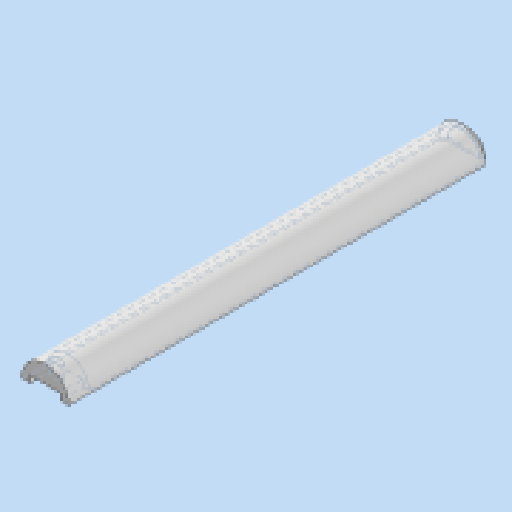
# Autodesk Inventor part: Shell_body_top
Saved by Autodesk Inventor 2024 (Build 280153000, 153)
## iProperties
Created: 2025-03-26
Part Number: Shell_body_top
Material: Generic
Document SubType Name: Modeling
Designer: XxPan
Density: 1 g/cm^3
Appearance: Default
Author: XxPan
Autodesk Inventor part; units mm, degrees
ref_plane "XY Plane" through (0, 0, 0) normal (0, 0, 1) x (1, 0, 0)
sketch "Sketch1" plane through (0, 0, 0) normal (0, 0, 1) x (1, 0, 0)
  arc A0 (8.5, 0) -> (-8.5, 0) centre (0, 0) ccw
  line L0 (-8.5, 0) -> (8.5, 0)
  dimension "d1" = 17
  constraints: 2 end point, 2 midpoint, 2 point on circle, 1 centre point, 1 coincident, 1 horizontal
  measures "d1" diameter of A0
extrude "Extrusion1" add sketch "Sketch1" against normal blind 150
chamfer "Chamfer1" distance 2 angle 45 1 edges at (0, 8.5, -150)
shell "Shell1" thickness 1 removed faces 2 at (2.1208, 1.8788, 0) at (-2.8333, 0, -98.6667)
ref_plane "Work Plane1" through (0, 2.3, 0) normal (0, 1, 0) x (-1, 0, 0)
sketch "Sketch2" plane through (0, 2.3, 0) normal (0, 1, 0) x (-1, 0, 0)
  line L0 (2, -3.4) -> (-2, -3.4) construction
  line L1 (2, -5) -> (-2, -5) construction
  line L2 (-2, -3.4) -> (-2, -5) construction
  line L3 (2, -5) -> (2, -3.4) construction
  line L4 (-2.1, -3.3) -> (2.1, -3.3)
  line L5 (2.1, -3.3) -> (2.1, -5.1)
  line L6 (2.1, -5.1) -> (-2.1, -5.1)
  line L7 (-2.1, -5.1) -> (-2.1, -3.3)
  line L8 (-7.5, 0) -> (7.5, 0) projected
  line L9 (-4, -8.16) -> (4, -8.16) projected
  line L10 (7.1386, 0) -> (7.1386, -8.16)
  line L11 (7.1386, 0) -> (15.2986, 0) construction
  line L12 (7.1386, -8.16) -> (4, -8.16)
  line L13 (-7.0941, 0) -> (1.0659, 0) construction
  line L14 (-7.1386, 0) -> (-7.1386, -8.16)
  line L15 (-7.1386, 0) -> (1.0214, 0) construction
  line L16 (-7.1386, -8.16) -> (-4, -8.16)
  point P0 (0, 0)
  dimension "d9" = 0.1
  dimension "d10" = 90
  dimension "d12" = 90
  constraints: 22 end point, 4 horizontal, 3 perpendicular, 1 point on line, 3 other
  measures "d9" distance between parallel lines of L0 L4
  measures "d10" angle of L10 L11
  measures "d12" angle of L14 L15
extrude "Extrusion2" add sketch "Sketch2" along normal up to surface
sketch "Sketch11" plane through (-6.5, 0, -150) normal (0, -1, 0) x (1, 0, 0)
  line L0 (1.5, 142.84) -> (1.5, 148.84) construction
  line L1 (11.5, 148.84) -> (11.5, 142.84) construction
  line L2 (-0.6386, 150) -> (13.6386, 150) construction
  line L3 (13.6386, 141.84) -> (-0.6386, 141.84) construction
  line L4 (-1, 2.4142) -> (-1, 150) projected
  line L5 (14, 150) -> (14, 2.4142) projected
  line L6 (-1, 150) -> (14, 150)
  line L7 (-1, 141.84) -> (14, 141.84)
  line L8 (1.3, 141.84) -> (1.3, 150)
  line L9 (11.7, 150) -> (11.7, 141.84)
  point P0 (6.5, 150)
  dimension "d62" = 0.2
  dimension "d63" = 0.2
  constraints: 8 end point, 6 point on line, 2 parallel, 2 perpendicular, 1 collinear
  measures "d62" distance between parallel lines of L0 L8
  measures "d63" distance between parallel lines of L1 L9
extrude "Extrusion10" add sketch "Sketch11" against normal up to surface (2.3 mm away) contours L4 L6 L8 L7 | L9 L6 L5 L7
chamfer "Chamfer2" distance 1 angle 45 4 edges at (2.1, 2.3, -4.2) (0, 2.3, -3.3) (0, 2.3, -5.1) (-2.1, 2.3, -4.2)
ref_plane "Work Plane2" through (0, 0, -12) normal (0, 0, 1) x (1, 0, 0)
sketch "Sketch3" plane through (0, 0, -12) normal (0, 0, 1) x (1, 0, 0)
  arc A0 (0.0865, 2.2483) -> (1.0622, -1.9835) centre (0, 0) ccw construction
  circle A1 centre (0, 0) radius 2.25
  line L0 (1.5, 1.6771) -> (1.5, 7.3485)
  line L1 (1.5, 1.6771) -> (9.5392, 1.6771) construction
  arc A2 (7.5, 0) -> (-7.5, 0) centre (0, 0) ccw projected
  line L2 (7.5, 0) -> (2.25, 0)
  line L3 (5.5, 0) -> (5.5, 5.099)
  line L4 (5.5, 0) -> (10.599, 0) construction
  dimension "d16" = 90
  dimension "d17" = 1.5
  dimension "d18" = 90
  dimension "d19" = 2
  constraints: 10 end point, 5 point on circle, 3 horizontal, 1 centre point, 1 coincident, 1 perpendicular, 1 point on line
  measures "d16" angle of L1 L0
  measures "d17" distance from line of L0 point (0, 0)
  measures "d18" angle of L4 L3
  measures "d19" distance from line of L2.start L3
extrude "Extrusion3" add sketch "Sketch3" against normal blind 7 contours A1 L0 A2 L3 L2
sketch "Sketch5" plane through (0, 0, 0) normal (0, 1, 0) x (-1, 0, 0)
  line L0 (-2.5, -78.4) -> (5.5, -78.4) projected
  line L1 (5.5, -77.4) -> (-2.5, -77.4) projected
  line L2 (2.5, -77.4) -> (2.5, -78.4)
  line L3 (7.5, -147.5858) -> (7.5, 0) projected
  line L4 (7.5, -77.4) -> (7.5, -78.4)
  line L5 (5.5, -77.4) -> (7.5, -77.4)
  line L6 (5.5, -78.4) -> (7.5, -78.4)
  point P0 (0, 0)
  dimension "d24" = 5
  constraints: 8 end point, 3 point on line, 2 perpendicular, 1 horizontal
  measures "d24" distance between parallel lines of L3 L2
extrude "Extrusion4" add sketch "Sketch5" along normal up to surface
sketch "Sketch6" plane through (0, 0, -150) normal (0, 0, -1) x (-1, 0, 0)
  arc A0 (1.625, -0.125) -> (-1.625, -0.125) centre (0, -0.125) ccw construction
  arc A1 (1.8207, 0) -> (-1.8207, 0) centre (0, -0.125) ccw
  line L0 (-6.5, 0) -> (6.5, 0) projected
  line L1 (-6.5, 0) -> (6.5, 0)
  point P0 (0, 0)
  point P1 (-1.8207, 0)
  point P2 (1.8207, 0)
  dimension "d27" = 0.2
  constraints: 2 end point, 2 point on circle, 2 point on line, 1 centre point, 1 collinear
  measures "d27" radial gap between concentric circles of A0 A1
extrude "Extrusion5" cut sketch "Sketch6" against normal up to surface (1 mm away)
ref_plane "Work Plane4" through (8.5, 0, 0) normal (1, 0, 0) x (0, 1, 0)
sketch "Sketch7" plane through (8.5, 0, 0) normal (1, 0, 0) x (0, 1, 0)
  line L0 (0, 0) -> (0, -148) projected
  line L1 (0, -123) -> (0, -133) construction
  line L2 (-2, -123) -> (-2, -133)
  line L3 (2, -133) -> (2, -123)
  arc A0 (2, -123) -> (-2, -123) centre (0, -123) ccw
  arc A1 (-2, -133) -> (2, -133) centre (0, -133) ccw
  line L4 (6.5, -150) -> (0, -150) projected
  point P0 (0, -128)
  point P1 (0, -121)
  point P2 (0, -135)
  dimension "d30" = 4
  dimension "d31" = 10
  dimension "d32" = 17
  constraints: 8 end point, 4 point on circle, 4 tangent, 2 centre point, 2 point on line, 1 midpoint, 1 parallel
  measures "d30" diameter of A1
  measures "d31" distance of L1.end L1.start
  measures "d32" distance from line of L4 L1.end
extrude "Extrusion6" cut sketch "Sketch7" against normal up to surface contours A0 L3 A1 L0
ref_plane "Work Plane5" through (0, 7, 0) normal (0, 1, 0) x (-1, 0, 0)
sketch "Sketch8" plane through (0, 7, 0) normal (0, 1, 0) x (-1, 0, 0)
  line L0 (-2.6926, -147.5858) -> (-2.6926, -47.5858)
  line L1 (-8.5, -148) -> (8.5, -148) projected
  line L2 (-2.6926, -147.5858) -> (97.3074, -147.5858) construction
  line L3 (2.6926, -147.5858) -> (2.6926, -47.5858)
  line L4 (2.6926, -147.5858) -> (102.6926, -147.5858) construction
  line L5 (-2.6926, -110) -> (2.6926, -110)
  line L6 (2.6926, -90) -> (-2.6926, -90)
  point P0 (0, 0)
  dimension "d36" = 100
  dimension "d37" = 90
  dimension "d38" = 100
  dimension "d39" = 90
  dimension "d40" = 20
  dimension "d41" = 38
  constraints: 12 end point, 4 perpendicular, 4 point on line, 3 horizontal, 1 vertical
  measures "d36" distance of L0.start L0.end
  measures "d37" angle of L2 L0
  measures "d38" distance of L3.start L3.end
  measures "d39" angle of L4 L3
  measures "d40" distance between parallel lines of L5 L6
  measures "d41" distance between parallel lines of L1 L5
extrude "Extrusion7" add sketch "Sketch8" along normal up to surface
sketch "Sketch9" plane through (0, 7, 0) normal (0, 1, 0) x (-1, 0, 0)
  arc A0 (-2.0001, -104.15) -> (2.0001, -104.15) centre (0, -104.15) ccw construction
  line L0 (-2.0001, -98.15) -> (-2.0001, -104.15) construction
  line L1 (2.0001, -104.15) -> (2.0001, -98.15) construction
  line L2 (2.2001, -98.15) -> (2.2001, -104.15)
  arc A1 (-2.2001, -104.15) -> (2.2001, -104.15) centre (0, -104.15) ccw
  line L3 (-2.2001, -104.15) -> (-2.2001, -98.15)
  arc A2 (2, -98.1324) -> (-2, -98.1324) centre (0, -98.15) ccw construction
  circle A3 centre (-0.0001, -96.25) radius 2 construction
  circle A4 centre (-0.0001, -96.25) radius 2.2
  line L4 (-2.2001, -98.15) -> (-2.2001, -96.25)
  line L5 (-2.2001, -98.15) -> (-1.2002, -98.15) construction
  line L6 (2.2001, -98.15) -> (2.1999, -96.2498)
  line L7 (2.2001, -98.15) -> (3.0189, -98.15) construction
  point P0 (0, 0)
  point P1 (2.1999, -96.25)
  dimension "d44" = 0.2
  dimension "d45" = 4
  dimension "d46" = 1.9
  dimension "d47" = 0.2
  dimension "d48" = 90
  constraints: 12 end point, 4 point on circle, 3 centre point, 2 horizontal, 2 tangent, 2 other
  measures "d44" radial gap between concentric circles of A0 A1
  measures "d45" diameter of A3
  measures "d46" distance of A3.centre A2.centre
  measures "d47" radial gap between concentric circles of A3 A4
  measures "d48" angle of L5 L4
extrude "Extrusion8" cut sketch "Sketch9" along normal up to surface
sketch "Sketch10" plane through (1.8207, 0, -150) normal (0, -1, 0) x (1, 0, 0)
  line L0 (4.2651, 1) -> (0, 1) projected
  line L1 (5.6793, 2.4142) -> (4.2651, 1) projected
  line L2 (5.6793, 15) -> (5.6793, 2.4142) projected
  line L3 (-3.6414, 1) -> (-7.9065, 1) projected
  line L4 (-7.9065, 1) -> (-9.3207, 2.4142) projected
  line L5 (-9.3207, 2.4142) -> (-9.3207, 71.6) projected
  line L6 (0, 1) -> (0, 3)
  line L7 (4.2651, 1) -> (-7.9065, 1) projected
  line L8 (0, 1) -> (2, 1) construction
  line L9 (0, 3) -> (5.6793, 3)
  line L10 (-5.3207, 1) -> (-5.3207, 3)
  line L11 (-5.3207, 3) -> (-9.3207, 3)
  point P0 (-1.8207, 150)
  dimension "d55" = 2
  dimension "d56" = 90
  dimension "d57" = 4
  constraints: 10 end point, 5 point on line, 4 perpendicular, 1 horizontal
  measures "d55" distance of L0.end L6.end
  measures "d56" angle of L8 L6
  measures "d57" distance between parallel lines of L5 L10
extrude "Extrusion9" add sketch "Sketch10" against normal up to surface
fillet "Fillet1" radius 2 8 edges at (0, 7.5, -8.16) (-2.5, 7.0711, -77.9) (-6.1237, 4.3301, -78.4) (-6.1237, 4.3301, -77.4) (5.9121, 4.6149, -147) (-6.4226, 3.873, -147) (-3.5, 6.6332, -147.2929) (1.8207, 7.2756, -147.2929)
body "Solid1"
